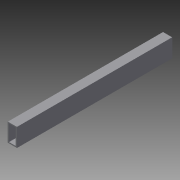
# Autodesk Inventor part: side 1
Saved by Autodesk Inventor 2013 (Build 170138000, 138)
## iProperties
Created: 2014-07-12
Part Number: side 1
Material: Generic
Document SubType Name: Modeling
Designer: admin
Density: 1 g/cm^3
Author: admin
Autodesk Inventor part; units mm, degrees
ref_plane "YZ Plane" through (0, 0, 0) normal (1, 0, 0) x (0, 1, 0)
ref_plane "XZ Plane" through (0, 0, 0) normal (0, 1, 0) x (-1, 0, 0)
ref_plane "XY Plane" through (0, 0, 0) normal (0, 0, 1) x (1, 0, 0)
sketch "Sketch1" plane through (0, 0, 0) normal (0, 0, 1) x (1, 0, 0)
  line L0 (9.525, 22.225) -> (9.525, -22.225)
  line L1 (9.525, -22.225) -> (-9.525, -22.225)
  line L2 (-9.525, -22.225) -> (-9.525, 22.225)
  line L3 (-9.525, 22.225) -> (9.525, 22.225)
  line L4 (12.7, 25.4) -> (-12.7, 25.4)
  line L5 (-12.7, 25.4) -> (-12.7, -25.4)
  line L6 (-12.7, -25.4) -> (12.7, -25.4)
  line L7 (12.7, -25.4) -> (12.7, 25.4)
  point P0 (0, 0)
  point P1 (0, 0)
  constraints: 16 end point
extrude "Extrusion1" add sketch "Sketch1" along normal blind 431.8
body "Solid1"
